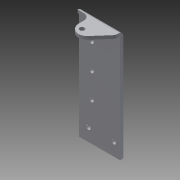
# Autodesk Inventor part: Pneumatic Piston Front Flange (Left Custom)
Saved by Autodesk Inventor 2014 (Build 180170000, 170)
## iProperties
Created: 2014-01-17
Part Number: Pneumatic Piston Front Flange (Left Custom)
Material: Aluminum 6061
Document SubType Name: Sheet Metal
Designer: Michael
Density: 2.71 g/cm^3
Sheet Metal Rule: Default
Appearance: Aluminum - Flat
Flat Pattern Width: 4.1275 cm
Flat Pattern Length: 13.1491 cm
Flat Pattern Area: 54.273 cm^2
Sheet Metal Width: 1.625 in
Sheet Metal Length: 5.177 in
Sheet Metal Area: 8.412 in^2
Author: Michael
Autodesk Inventor part; units mm, degrees
note: some values were not read from the file. Chosen so that the rebuilt part matches the saved one: flange form of "Plate2". Left out: dimensions or parameters whose unit could not be read.
ref_plane "YZ Plane" through (0, 0, 0) normal (1, 0, 0) x (0, 1, 0)
ref_plane "XZ Plane" through (0, 0, 0) normal (0, 1, 0) x (-1, 0, 0)
ref_plane "XY Plane" through (0, 0, 0) normal (0, 0, 1) x (1, 0, 0)
sketch "Sketch1 outline for Plate1" plane through (0, 0, 0) normal (0, 0, 1) x (1, 0, 0)
  line L0 (0, 106.3625) -> (0, 0)
  line L1 (41.275, 106.3625) -> (0, 106.3625)
  line L2 (0, 0) -> (41.275, 0)
  line L3 (41.275, 0) -> (41.275, 106.3625)
  circle A0 centre (9.525, 12.7) radius 2.0701
  circle A1 centre (12.7, 38.1) radius 2.0701
  circle A2 centre (34.925, 12.7) radius 2.0701
  circle A3 centre (12.7, 63.5) radius 2.0701
  circle A4 centre (12.7, 88.9) radius 2.0701
extrude "Plate1" add sketch "Sketch1 outline for Plate1" along normal blind 3.175
sketch "Sketch2" plane through (0, 107.6325, 4.445) normal (0, 1, 0) x (-1, 0, 0)
  line L0 (-41.275, 0) -> (0, 0)
  line L1 (0, 0) -> (0, 20.955)
  line L2 (0, 20.955) -> (-41.275, 20.955)
  line L3 (-41.275, 20.955) -> (-41.275, 0)
  constraints: 6 end point, 1 horizontal, 1 perpendicular, 1 vertical
edge flange "Flange1" height 25.4 angle 90 thickness 3.175 bend radius 1.27 thickness toward (0, 1, 0) relief tear relief width 3.175 relief depth 1.5875 edges at (20.6375, 106.3625, 3.175) wall of the first edge with corners at (41.275, 107.6325, 4.445) (0, 107.6325, 4.445) (0, 107.6325, 25.4) (41.275, 107.6325, 25.4)
bend "Bend1"
corner "Corner1"
sketch "Sketch1" plane through (0, 0, 0) normal (0, 0, 1) x (1, 0, 0)
  line L0 (110.551814, -41.275) -> (0, -41.275)
  line L1 (110.551814, -34.925) -> (110.551814, -41.275)
  line L2 (0, 0) -> (111.304505, 0)
  line L3 (106.3625, 0) -> (110.551814, 0)
  line L4 (110.551814, 0) -> (110.551814, -3.175)
  line L5 (110.551814, -3.175) -> (106.3625, -3.175)
  line L6 (106.3625, -3.175) -> (106.3625, 0)
  line L7 (106.3625, 0) -> (106.3625, -41.275)
  line L8 (110.551814, 0) -> (110.551814, -34.925)
  line L9 (106.3625, -38.1) -> (110.551814, -38.1)
  line L10 (110.551814, -38.1) -> (110.551814, -41.275)
  line L11 (110.551814, -41.275) -> (106.3625, -41.275)
  line L12 (106.3625, -41.275) -> (106.3625, -38.1)
  dimension "d6" = 25.4
  dimension "d22" = 12.7
  dimension "d36" = 6.35
  dimension "d38" = 12.7
  dimension "d39" = 38.1
  dimension "d42" = 25.4
  measures "d22" distance between parallel lines of L0 L4
sketch "Sketch4" plane through (0, 110.8075, 25.4) normal (0, 1, 0) x (1, 0, 0)
  line L0 (41.275, 0) -> (0, 0)
  circle A0 centre (19.05, 6.35) radius 2.3749
  line L1 (0, 0) -> (0, 20.955)
  line L2 (0, 20.955) -> (41.275, 20.955)
  line L3 (41.275, 20.955) -> (41.275, 21.413463)
  line L4 (21.135301, 0) -> (22.225, 0)
  line L5 (0, 0) -> (0, 20.955)
  line L6 (41.275, 20.955) -> (0, 20.955)
  line L7 (41.275, 20.955) -> (41.275, 17.78)
  line L8 (41.275, 17.78) -> (28.240357, 3.1812)
  line L9 (12.7, 9.525) -> (12.7, 20.955)
  arc A1 (12.7, 9.525) -> (21.68015, 0.015596) centre (22.225, 9.525) ccw
  arc A2 (21.68015, 0.015596) -> (28.240357, 3.1812) centre (21.135301, 9.525) ccw
  line L10 (41.275, 20.955) -> (41.275, 0)
  line L11 (0, 0) -> (41.275, 0)
  line L12 (41.275, 0) -> (41.275, 20.955)
  point P0 (0, 25.4)
  point P1 (12.7, 0)
  point P2 (25.4, 0)
  point P3 (12.7, 0)
  dimension "d28" = 4.7498
  dimension "d29" = 6.35
  dimension "d34" = 19.05
  dimension "d47" = 3.175
  dimension "d48" = 6.35
  dimension "d49" = 6.35
  dimension "d50" = 9.525
  constraints: 18 end point, 10 point on line, 4 point on circle, 4 tangent, 3 centre point, 3 perpendicular, 2 parallel, 1 collinear, 1 equal radius, 1 horizontal, 1 vertical
  measures "d28" diameter of A0
  measures "d29" distance from line of L0 A0.centre
  measures "d34" distance from line of L1 A0.centre
  measures "d47" distance of L7.end L6.start
  measures "d48" distance from line of A0.centre L9
  measures "d49" horizontal distance of point (25.4, 0) A0.centre
  measures "d50" radius of A1
extrude "Cut3" cut sketch "Sketch4" against normal blind 3.175 contours L0 L1 L2 L9 A1 A2 L8 L10 | A0
fillet "Fillet3" radius 6.35 2 edges at (41.275, 109.22, 7.62) (12.7, 109.22, 4.445)
equation "\"d51\" = Thickness"
equation "\"d12\" = BendReliefWidth"
equation "\"d13\" = BendReliefDepth"
equation "\"d14\" = MinimumRemnant"
equation "\"d15\" = BendRadius"
equation "\"d19\" = CornerReliefSize"
equation "\"d20\" = GapSize"
equation "\"d21\" = JacobiRadiusSize"
equation "\"BendRadius\" = Thickness"
equation "\"BendReliefWidth\" = Thickness"
equation "\"BendReliefDepth\" = 0.5 * Thickness"
equation "\"CornerReliefSize\" = 4 * Thickness"
equation "\"MinimumRemnant\" = 2 * Thickness"
equation "\"TransitionRadius\" = BendRadius"
equation "\"JacobiRadiusSize\" = BendRadius"
equation "\"GapSize\" = Thickness"
equation "\"d11\" = BendRadius"
equation "\"Thickness\" = 3.175"
body "Solid1"
